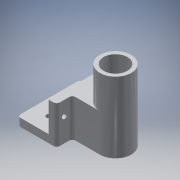
# Autodesk Inventor part: flange
Saved by Autodesk Inventor 2018 (Build 220112000, 112)
## iProperties
Part Number: flange
Material: ABS-Kunststoff
Document SubType Name: Modeling
Designer: Till
Density: 1.06 g/cm^3
Appearance: Glatt - weiß
Author: Till
Autodesk Inventor part; units mm, degrees
note: some values were not read from the file. Chosen so that the rebuilt part matches the saved one: second side of "Extrusion5".
ref_plane "YZ Plane" through (0, 0, 0) normal (1, 0, 0) x (0, 1, 0)
ref_plane "XZ Plane" through (0, 0, 0) normal (0, 1, 0) x (-1, 0, 0)
ref_plane "XY Plane" through (0, 0, 0) normal (0, 0, 1) x (1, 0, 0)
sketch "Skizze1" plane through (0, 0, 0) normal (0, 0, 1) x (1, 0, 0)
  circle A0 centre (0, 0) radius 7.6
  line L0 (-22.5, 20) -> (-22.5, -20)
  line L1 (-22.5, -20) -> (-17.5, -20)
  line L2 (-17.5, -20) -> (-17.5, -10)
  line L3 (-22.5, 20) -> (-17.5, 20)
  line L4 (-17.5, 20) -> (-17.5, 10)
  line L5 (-17.5, 10) -> (0, 10)
  line L6 (-17.5, -10) -> (0, -10)
  arc A1 (0, -10) -> (0, 10) centre (0, 0) ccw
  dimension "d0" = 15.2
  dimension "d23" = 5
  dimension "d24" = 10
  dimension "d25" = 5
  dimension "d26" = 10
  dimension "d27" = 40
  dimension "d28" = 20
  dimension "d38" = 22.5
  constraints: 14 end point, 3 horizontal, 2 centre point, 2 coincident, 2 perpendicular, 2 point on circle, 1 parallel, 1 vertical
  measures "d0" diameter of A0
  measures "d23" distance of L0.end L1.end
  measures "d24" distance of L1.end L2.end
  measures "d25" distance of L0.start L3.end
  measures "d26" distance of L3.end L4.end
  measures "d27" distance of L0.end L0.start
  measures "d28" vertical distance of point (0, 0) L0.end
  measures "d38" distance from line of point (0, 0) L0
extrude "Extrusion1" add sketch "Skizze1" along normal blind 24
sketch "Skizze2" plane through (-22.5, -20, 0) normal (-1, 0, 0) x (0, 0, 1)
  line L0 (0, 40) -> (0, 0) projected
  line L1 (0, 0) -> (24, 0) projected
  line L2 (0, 40) -> (5, 40)
  line L3 (5, 40) -> (5, 0)
  line L4 (5, 0) -> (0, 0)
  line L5 (0, 0) -> (0, 40)
  point P0 (0, 20)
  dimension "d12" = 5
  constraints: 8 end point, 2 parallel, 1 horizontal, 1 perpendicular, 1 point on line
  measures "d12" distance of L3.end L4.end
extrude "Extrusion2" add sketch "Skizze2" along normal blind 20
sketch "Skizze3" plane through (-22.5, -20, 5) normal (0, 0, 1) x (1, 0, 0)
  circle A0 centre (-10, 30) radius 1.6
  line L0 (0, 40) -> (-20, 40) projected
  line L1 (-20, 0) -> (-20, 40) projected
  circle A1 centre (-10, 10) radius 1.6
  line L2 (0, 0) -> (-20, 0) projected
  point P0 (22.5, 20)
  dimension "d15" = 3.2
  dimension "d16" = 10
  dimension "d17" = 10
  dimension "d18" = 3.2
  dimension "d19" = 10
  dimension "d20" = 10
  constraints: 2 centre point
  measures "d15" diameter of A0
  measures "d16" distance from line of L0 A0.centre
  measures "d17" distance from line of L1 A0.centre
  measures "d18" diameter of A1
  measures "d19" distance from line of L1 A1.centre
  measures "d20" distance from line of L2 A1.centre
extrude "Extrusion3" cut sketch "Skizze3" against normal through all
fillet "Rundung1" radius 2 6 edges at (-17.5, -10, 12) (-17.5, 10, 12) (-17.5, 20, 12) (-17.5, -20, 12) (-42.5, -20, 2.5) (-42.5, 20, 2.5)
sketch "Skizze4" plane through (-17.5, -18, 0) normal (1, 0, 0) x (0, 0, -1)
  circle A0 centre (-15, 3) radius 1.6
  circle A1 centre (-15, 33) radius 1.6
  line L0 (0, 0) -> (0, 6) projected
  line L1 (-24, -2) -> (0, -2) projected
  line L2 (-5, 38) -> (-24, 38) projected
  point P0 (0, 18)
  dimension "d30" = 3.2
  dimension "d31" = 3.2
  dimension "d32" = 15
  dimension "d33" = 5
  dimension "d34" = 15
  dimension "d35" = 5
  constraints: 2 centre point
  measures "d30" diameter of A0
  measures "d31" diameter of A1
  measures "d32" distance from line of L0 A0.centre
  measures "d33" distance from line of L1 A0.centre
  measures "d34" distance from line of L0 A1.centre
  measures "d35" distance from line of L2 A1.centre
extrude "Extrusion4" cut sketch "Skizze4" against normal through all
sketch "Skizze5" plane through (0, 0, 24) normal (0, 0, 1) x (1, 0, 0)
  circle A0 centre (0, 0) radius 7.6
  circle A1 centre (0, 0) radius 10
  constraints: 2 centre point, 2 coincident
extrude "Extrusion5" add sketch "Skizze5" along normal blind 21
